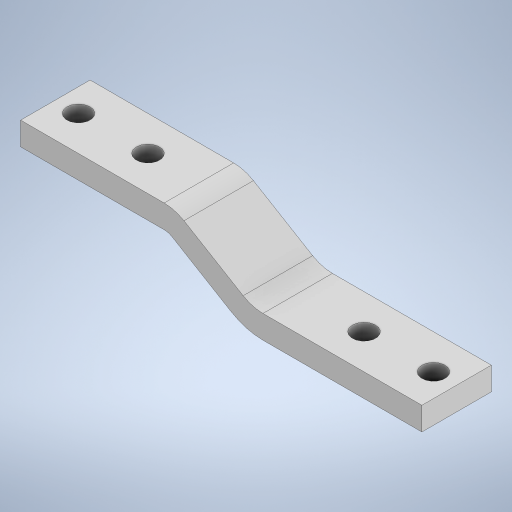
# Autodesk Inventor part: Hudson 1-68
Saved by Autodesk Inventor 2024.2 (Build 282272000, 272)
## iProperties
Created: 2024-10-10
Part Number: Hudson 1-68
Material: Generic
Document SubType Name: Modeling
Designer: Precisión-12
Density: 1 g/cm^3
Appearance: Default
Author: Precisión-12
Autodesk Inventor part; units mm, degrees
ref_plane "YZ Plane" through (0, 0, 0) normal (1, 0, 0) x (0, 1, 0)
ref_plane "XZ Plane" through (0, 0, 0) normal (0, 1, 0) x (-1, 0, 0)
sketch "Sketch1" plane through (0, 0, 0) normal (0, 0, 1) x (1, 0, 0)
  line L0 (0, 0) -> (0, 3)
  line L1 (0, 0) -> (0, 40.1132) construction
  arc A0 (-23.165, 3.7081) -> (-20.6, 3) centre (-20.6, 8) ccw
  line L2 (0, 3) -> (-20.6, 3)
  line L3 (0, 0) -> (-20.6, 0)
  arc A1 (-24.704, 1.1329) -> (-20.6, 0) centre (-20.6, 8) ccw
  line L4 (-52, 6) -> (-33.4, 6)
  line L5 (-52, 6) -> (-52, 9)
  line L6 (-52, 9) -> (-33.4, 9)
  circle A2 centre (-33.4, 4) radius 2
  arc A3 (-30.835, 8.2919) -> (-37.9826, 6) centre (-33.4, 4) ccw
  line L7 (-32.374, 5.7168) -> (-24.704, 1.1329)
  line L8 (-30.835, 8.2919) -> (-23.165, 3.7081)
  dimension "d9" = 4
  dimension "d0" = 20.6
  dimension "d2" = 10
  dimension "d3" = 3
  dimension "d4" = 6
  dimension "d5" = 12.8
  dimension "d6" = 3
  dimension "d7" = 18.6
  dimension "d8" = 18.6
  dimension "d10" = 10
  dimension "d11" = 12.8
  constraints: 18 end point, 6 point on circle, 5 tangent, 4 horizontal, 3 centre point, 3 vertical, 2 coincident, 1 perpendicular, 1 point on line, 4 other
  measures "d0" distance from line of L1 A0.centre
  measures "d2" diameter of A0
  measures "d3" distance between parallel lines of L3 L2
  measures "d4" distance between parallel lines of L3 L4
  measures "d5" horizontal distance of A0.centre L4.end
  measures "d6" distance between parallel lines of L4 L6
  measures "d7" distance of L5.end L6.end
  measures "d8" distance of L4.start L4.end
  measures "d10" diameter of A3
  measures "d11" horizontal distance of A0.centre point (-33.4, 4)
extrude "Extrusion1" add sketch "Sketch1" along normal mid plane 9 contours L3 A1 L7 A2 L4 A3 L8 A0 L2 L0 | A3 L4 L5 L6
ref_plane "Work Plane1" through (-52, 11, 4.5) normal (0, 1, 0) x (1, 0, 0)
sketch "Sketch2" plane through (-52, 11, 4.5) normal (0, 1, 0) x (1, 0, 0)
  line L0 (0, 9) -> (0, 0) projected
  line L1 (31.4, 9) -> (52, 9) projected
  line L2 (18.6, 9) -> (0, 9) projected
  line L3 (3, 9) -> (3, 0) construction
  line L4 (18.6, 0) -> (0, 0) projected
  line L5 (12, 9) -> (12, 0) construction
  line L6 (49, 9) -> (49, 0) construction
  line L7 (31.4, 0) -> (52, 0) projected
  line L8 (0, 4.5) -> (52, 4.5) construction
  line L9 (52, 9) -> (52, 0) projected
  line L10 (40, 9) -> (40, 0) construction
  circle A0 centre (3, 4.5) radius 1.5
  circle A1 centre (12, 4.5) radius 1.5
  circle A2 centre (40, 4.5) radius 1.5
  circle A3 centre (49, 4.5) radius 1.5
  dimension "d15" = 3
  dimension "d16" = 9
  dimension "d17" = 3
  dimension "d18" = 9
  dimension "d19" = 3
  dimension "d20" = 3
  dimension "d21" = 3
  dimension "d22" = 3
  constraints: 10 end point, 8 point on line, 5 midpoint, 4 centre point, 2 vertical, 1 horizontal, 1 perpendicular
  measures "d15" distance between parallel lines of L0 L3
  measures "d16" distance between parallel lines of L3 L5
  measures "d17" distance between parallel lines of L9 L6
  measures "d18" distance between parallel lines of L6 L10
  measures "d19" diameter of A0
  measures "d20" diameter of A1
  measures "d21" diameter of A2
  measures "d22" diameter of A3
hole "Hole1" at (-12, 11, 0) at (-3, 11, 0) at (-40, 11, 0) at (-49, 11, 0) direction (0, -1, 0) diameter 3 end through all
equation "\"d8\" = d7"
body "Solid1"
